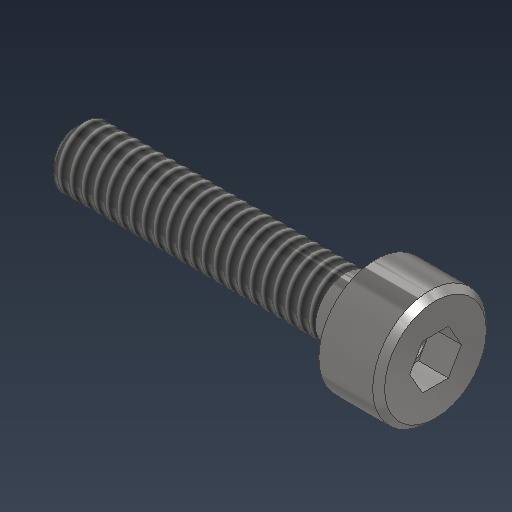
# Autodesk Inventor part: CB2-10
Saved by Autodesk Inventor 2021 (Build 250183000, 183)
## iProperties
Category: PARTsolutions
Company: MISUMI
Part Number: CB2-10
Material: 鋼、炭素鋼
Catalog Web Link: www.cadenas.de
Description: CB-Hexagon Socket Head Cap Screws
Vendor: MISUMI
Document SubType Name: Modeling
Designer: partserver
Manufacturer: MISUMI
Mass: 0.405272 g
Surface Area: 1.12216 cm^2
Volume: 0.0516271 cm^3
Density: 7.85 g/cm^3
Appearance: 半つや出し
PSOL_IDENT_0: {$CADENAS_DATA\23d-libs\misumi\metric\27_screws_nuts\cb_fa.prj},150 {VTYP=3D},{NB=CB2-10},{LINA=CB2-
PSOL_IDENT_1: 10},{NN=CB},{DATE=09.09.2019 15:27:56},{GEOMDATE=17.02.2014 00:00:00},{VERSION=},{LINEID=10},{WBVAR=
PSOL_IDENT_2: L},{WBNUMERIC=L}  {NB=CB2-10},{LINA=CB2-10},{KT=DUMMY},{PN=CB2-10},{MAT=4137 Steel},{HARD=38~43HRC},
PSOL_IDENT_3: {ST=Black Oxide},{M=2},{L=10},{LL=Full Thread},{L1=60},{TYPE=CB},{M1=2.000},{L0=4,5,6,8,10,12,15},{N
PSOL_IDENT_4: DM=2},{KDM=1.508532},{MP=2x0.4},{P=0.4},{A=3.8},{E=2.0},{B=1.5},{V=0.2}
NB: CB2-10
NN: CB
NT: Hexagon Socket Head Cap Screws
NBSYN: $PN.
LINA: CB2-10
CATALOG: Misumi
PN: CB2-10
MAT: 4137 Steel
HARD: 38~43HRC
ST: Black Oxide
M: 2
L: 10
LL: Full Thread
MP: 2x0.4
A: 3.8
E: 2
B: 1.5
SUPPLIER: MISUMI
ARTICLENO: CB2-10
BOMINFO: CB2-10
CREATOR: CADENAS GmbH
購入先: ミスミ
在庫数: 0.0
Title: CB2-10
Author: Cadenas PARTsolutions
Comments: Hexagon Socket Head Cap Screws
Autodesk Inventor part; units mm, degrees
sketch "Sketch_1" plane through (0, 0, 0) normal (0, 0, 1) x (1, 0, 0)
  line L0 (10, 0) -> (-2, 0)
  line L1 (-2, 0) -> (-2, 1.7)
  line L2 (-2, 1.7) -> (-1.8, 1.9)
  line L3 (-1.8, 1.9) -> (0, 1.9)
  line L4 (0, 1.9) -> (0, 1)
  line L5 (0, 1) -> (9.7545, 1)
  line L6 (9.7545, 1) -> (10, 0.7545)
  line L7 (10, 0.7545) -> (10, 0)
  line L8 (10, 0) -> (-2, 0)
  constraints: 18 end point
revolve "Revolution1" add sketch "Sketch_1" angle 360 about axis through (10, 0, 0) along (1, 0, 0)
thread "Thread1" size "M2x0.4" class "6g" standard "ISO Metric profile" length 8.7545
sketch "Sketch2" plane through (-2, 0, 0) normal (-1, 0, 0) x (0, 0, 1)
  point P0 (0, 0)
hole "Hole1" at (-2, 0, 0) direction (1, 0, 0) diameter 1.5 depth 1 tip angle 150
sketch "Sketch_3" plane through (-2, 0, 0) normal (1, 0, 0) x (0, 0, -1)
  line L0 (-0.75, -0.433) -> (0, -0.866)
  line L1 (0, -0.866) -> (0.75, -0.433)
  line L2 (0.75, -0.433) -> (0.75, 0.433)
  line L3 (0.75, 0.433) -> (0, 0.866)
  line L4 (0, 0.866) -> (-0.75, 0.433)
  line L5 (-0.75, 0.433) -> (-0.75, -0.433)
  constraints: 12 end point
extrude "Extrusion1" cut sketch "Sketch_3" along normal blind 1
ref_plane "bolt_to_nut_XY" through (10, 0, 0) normal (1, 0, 0) x (0, 0, -1)
ref_plane "bolt_to_nut_YZ" through (10, 0, 0) normal (0, 0, -1) x (0, 1, 0)
ref_plane "bolt_to_nut_ZX" through (10, 0, 0) normal (0, 1, 0) x (1, 0, 0)
ref_plane "screw1_XY" through (0, 0, 0) normal (1, 0, 0) x (0, 0, -1)
ref_plane "screw1_YZ" through (0, 0, 0) normal (0, 0, -1) x (0, 1, 0)
ref_plane "screw1_ZX" through (0, 0, 0) normal (0, 1, 0) x (1, 0, 0)
body "Solid1"
